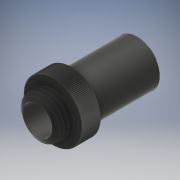
# Autodesk Inventor part: Objetivo 600x
Saved by Autodesk Inventor 2018 (Build 220112000, 112)
## iProperties
Created: 2018-06-04
Part Number: Objetivo 600x
Material: Acetal Resin, Black
Document SubType Name: Modeling
Designer: Michel Gordillo
Density: 1.425 g/cm^3
Appearance: Smooth - Black
Author: Michel Gordillo
Autodesk Inventor part; units mm, degrees
ref_plane "YZ Plane" through (0, 0, 0) normal (1, 0, 0) x (0, 1, 0)
ref_plane "XZ Plane" through (0, 0, 0) normal (0, 1, 0) x (-1, 0, 0)
sketch "Sketch1" plane through (0, 0, 0) normal (0, 0, 1) x (1, 0, 0)
  line L0 (0, 0) -> (4.5, 0)
  line L1 (4.5, 0) -> (4.5, 3.5)
  line L2 (4.5, 3.5) -> (6.5, 3.5)
  line L3 (6.5, 3.5) -> (6.5, 7.5)
  line L4 (5, 8.5) -> (5, 8.5)
  line L5 (5, 8.5) -> (5, 22)
  line L6 (3, 23.5) -> (0, 23.5)
  line L7 (0, 23.5) -> (0, 0)
  line L8 (6.5, 7.5) -> (5, 8.5)
  line L9 (5, 22) -> (3, 23.5)
  point P0 (6.5, 8.5)
  point P1 (5, 23.5)
  dimension "d0" = 4.5
  dimension "d1" = 2
  dimension "d2" = 5
  dimension "d3" = 15
  dimension "d4" = 5
  dimension "d5" = 1
  dimension "d6" = 1.5
  dimension "d7" = 1.5
  dimension "d8" = 2
  dimension "d9" = 3.5
  constraints: 20 end point, 6 perpendicular, 4 point on line, 2 horizontal
  measures "d0" distance of L0.start L0.end
  measures "d1" distance of L1.end L2.end
  measures "d2" distance of L2.end point (6.5, 8.5)
  measures "d3" distance of L4.end point (5, 23.5)
  measures "d4" distance of point (5, 23.5) L6.end
  measures "d5" distance of L3.end point (6.5, 8.5)
  measures "d6" distance of L4.start point (6.5, 8.5)
  measures "d7" distance of L5.end point (5, 23.5)
  measures "d8" distance of L6.start point (5, 23.5)
  measures "d9" distance of L0.end L1.end
revolve "Revolution1" add sketch "Sketch1" angle 360 about axis through (0, 23.5, 0) along (0, -1, 0)
ref_plane "Work Plane1" through (0, 0, 0) normal (0, 0, 1) x (1, 0, 0)
sketch "Sketch2" plane through (0, 0, 0) normal (0, 0, 1) x (1, 0, 0)
  line L0 (-4.5, 3.5) -> (4.5, 3.5) projected
  line L1 (4.5, 3.5) -> (4.5, 4.5)
  line L2 (4.5, 4.5) -> (3.634, 4)
  line L3 (3.634, 4) -> (4.5, 3.5)
  point P0 (0, 0)
  dimension "d12" = 1
  dimension "d13" = 1
  dimension "d14" = 1
  constraints: 6 end point, 1 vertical
  measures "d12" distance of L0.end L1.end
  measures "d13" distance of L1.end L2.end
  measures "d14" distance of L2.end L0.end
coil "Coil1" sketch "Sketch2" operation cut axis through (0, -10, 0) along (0, -1, 0) pitch 1 turns 5 hand right
sketch "Sketch3" plane through (0, 3.5, 0) normal (0, -1, 0) x (1, 0, 0)
  circle A0 centre (0, 0) radius 5
  constraints: 1 centre point, 1 coincident
extrude "Extrusion1" add sketch "Sketch3" against normal blind 3
sketch "Sketch4" plane through (0, 0, 0) normal (0, 0, 1) x (1, 0, 0)
  line L0 (-3.1015, -0.0129) -> (-4.5944, 0.849)
  line L1 (-4.5944, 0.849) -> (-4.5944, -0.5977)
  line L2 (-4.5944, -0.5977) -> (-3.1015, -0.5977)
  line L3 (-3.1015, -0.5977) -> (-3.1015, -0.0129)
  line L4 (0, -5.4172) -> (0, 28.3195) projected
  point P0 (0, 0)
  dimension "d25" = 30
  constraints: 8 end point, 2 perpendicular, 1 vertical
  measures "d25" angle of L2 L0
revolve "Revolution2" cut sketch "Sketch4" angle 360 about axis through (0, -10, 0) along (0, 1, 0)
sketch "Sketch5" plane through (0, 0, 0) normal (0, -1, 0) x (1, 0, 0)
  circle A0 centre (0, 0) radius 3.25
  dimension "d27" = 6.5
  constraints: 1 centre point, 1 coincident
  measures "d27" diameter of A0
extrude "Extrusion2" cut sketch "Sketch5" against normal blind 14
sketch "Sketch6" plane through (0, 14, 0) normal (0, -1, 0) x (1, 0, 0)
  circle A0 centre (0, 0) radius 2.25
  dimension "d30" = 4.5
  constraints: 1 centre point, 1 coincident
  measures "d30" diameter of A0
extrude "Extrusion3" cut sketch "Sketch6" against normal blind 4
sketch "Sketch7" plane through (0, 23.5, 0) normal (0, 1, 0) x (1, 0, 0)
  circle A0 centre (0, 0) radius 1
  dimension "d33" = 2
  constraints: 1 centre point, 1 coincident
  measures "d33" diameter of A0
extrude "Extrusion4" cut sketch "Sketch7" against normal through all
chamfer "Chamfer1" distance 0.2 angle 45 1 edges at (-1, 23.5, 0)
sketch "Sketch8" plane through (0, 3.5, 0) normal (0, -1, 0) x (1, 0, 0)
  line L0 (0, 0) -> (0.2835, -6.4938)
  circle A0 centre (0, 0) radius 6.5 projected
  line L1 (0, 0) -> (6.5, 0) construction
  line L2 (0.2835, -6.4938) -> (0.1293, -6.2517)
  line L3 (0.1293, -6.2517) -> (0, -6.5)
  dimension "d39" = 87.5
  dimension "d40" = 30
  dimension "d41" = 60
  constraints: 8 end point, 2 point on circle, 1 equal length, 1 horizontal
  measures "d39" angle of L0 L1
  measures "d40" angle of L0 L2
  measures "d41" angle of L2 L3
extrude "Extrusion5" cut sketch "Sketch8" against normal up to next contours L3 L2 A0 picked at (0.2006, -6.4143)
pattern_circular "Circular Pattern1" count 144 over 360 about axis through (0, 5.5, 0) along (0, -1, 0) of "Extrusion5"
body "Solid1"
